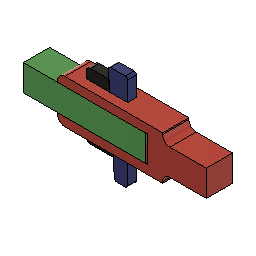
cotter and gip (Autodesk Fusion 360 design; units mm, degrees)
Autodesk Fusion 360 part; units mm, degrees
sketch "Sketch1" plane through (0, 0, 0) normal (0, 0, 1) x (1, 0, 0)
  line L0 (0, 0) -> (0, 20)
  line L1 (0, 20) -> (-170, 20)
  line L2 (-170, 20) -> (-170, -16)
  line L3 (-170, -16) -> (0, -16)
  line L4 (0, -16) -> (0, 0)
  line L5 (0, -16) -> (-39, -16)
  line L6 (83.0613, 20) -> (203.0613, 20)
  line L7 (203.0613, 20) -> (203.0613, -16)
  line L8 (203.0613, -16) -> (83.0613, -16)
  line L9 (83.0613, 20) -> (83.0613, 22)
  line L10 (83.0613, -16) -> (83.0613, -18)
  line L11 (83.0613, -28) -> (83.0613, -25)
  line L12 (93.0613, 32) -> (227.0613, 32)
  line L13 (227.0613, 32) -> (227.0613, 30)
  line L14 (227.0613, -28) -> (93.0613, -28)
  line L15 (237.0613, 20) -> (287.0613, 20)
  line L16 (237.0613, -16) -> (287.0613, -16)
  line L17 (287.0613, -16) -> (287.0613, 20)
  arc A0 (227.0613, 30) -> (237.0613, 20) centre (237.0613, 30) ccw
  line L18 (227.0613, -28) -> (227.0613, -26)
  arc A1 (237.0613, -16) -> (227.0613, -26) centre (237.0613, -26) ccw
  arc A2 (93.0613, 32) -> (83.0613, 22) centre (93.0613, 22) ccw
  arc A3 (83.0613, -18) -> (93.0613, -28) centre (93.0613, -18) ccw
  point P0 (83.0613, 32)
  point P1 (227.0613, 20)
  point P2 (227.0613, -16)
  dimension "d1" = 36
  dimension "d2" = 170
  dimension "d3" = 39
  dimension "d11" = 36
  dimension "d13" = 120
  dimension "d14" = 36
  dimension "d15" = 12
  dimension "d16" = 12
  dimension "d17" = 144
  dimension "d18" = 60
  dimension "d20" = 60
  dimension "d21" = 10
  dimension "d22" = 10
  dimension "d23" = 10
  dimension "d24" = 10
  constraint coincident L0.start L4.end
  constraint vertical L0
  constraint perpendicular L0 L1
  constraint perpendicular L1 L2
  constraint perpendicular L2 L3
  constraint perpendicular L3 L4
  constraint coincident L3 L5.end
  constraint perpendicular L6 L7
  constraint perpendicular L6 L9
  constraint perpendicular L8 L10
  constraint coincident L10 L11.end
  constraint perpendicular L9 L12
  constraint perpendicular L12 L13
  constraint perpendicular L10 L14
  constraint coincident L13 P1
  constraint perpendicular L13 L15
  constraint coincident L13 P2
  constraint perpendicular L13 L16
  constraint perpendicular L15 L17
  constraint coincident L14.start L13
  constraint coincident P1 L15
  constraint tangent L13 A0
  constraint tangent L15 A0
  constraint coincident P2 L18
  constraint coincident P2 L16
  constraint tangent L18 A1
  constraint tangent L16 A1
  constraint coincident P0 L9
  constraint coincident P0 L12
  constraint tangent L9 A2
  constraint tangent L12 A2
  constraint coincident L11.start L10
  constraint tangent L10 A3
  constraint tangent L14 A3
  measures "d1" distance of L1.end L2.end
  measures "d2" distance of L0.end L1.end
  measures "d3" distance of L3.end L5.end
  measures "d11" distance of L8.end L6.start
  measures "d13" distance of L6.start L6.end
  measures "d14" distance of L6.end L7.end
  measures "d15" distance of L6.start P0
  measures "d16" distance of L8.end L11.start
  measures "d17" distance of P0 L12.end
  measures "d18" distance of L12.end L14.start
  measures "d20" distance of P2 L16.end
  measures "d21" radius of A0
  measures "d22" radius of A1
  measures "d23" radius of A2
  measures "d24" radius of A3
extrude "Extrude1" add sketch "Sketch1" along normal mid plane 36 makes body 1 at (-113.3333, -16, 6) makes body 2 at (270.3947, -4, 18)
sketch "Sketch2" plane through (0, 20, 0) normal (0, 1, 0) x (-1, 0, 0)
  line L0 (170, -18) -> (170, 18)
  line L1 (170, 18) -> (0, 18)
  line L2 (0, 18) -> (0, -18)
  line L3 (0, -18) -> (170, -18)
  line L4 (0, 18) -> (170, 18)
  line L5 (170, -18) -> (170, 18)
  line L6 (170, -18) -> (0, -18)
  line L7 (0, -18) -> (0, 18)
  line L8 (-227.0613, 18) -> (-93.0613, 18)
  line L9 (-93.0613, -18) -> (-93.0613, 18)
  line L10 (-93.0613, -18) -> (-227.0613, -18)
  line L11 (-227.0613, -18) -> (-227.0613, 18)
  line L12 (39, -6) -> (39, 6)
  line L13 (39, 6) -> (84, 6)
  line L14 (84, 6) -> (84, -6)
  line L15 (84, -6) -> (39, -6)
  line L16 (-93.0613, -18) -> (-122.0613, -18)
  line L17 (-122.0613, -18) -> (-122.0613, -6)
  line L18 (-122.0613, -6) -> (-122.0613, 6)
  line L19 (-122.0613, 6) -> (-167.0613, 6)
  line L20 (-167.0613, 6) -> (-167.0613, -6)
  line L21 (-167.0613, -6) -> (-122.0613, -6)
  dimension "d29" = 12
  dimension "d30" = 45
  dimension "d31" = 12
  dimension "d32" = 29
  dimension "d33" = 12
  dimension "d34" = 12
  dimension "d35" = 45
  dimension "d36" = 12
  constraint perpendicular L13 L14
  constraint coincident L9.start L10.start
  constraint perpendicular L9 L16
  constraint perpendicular L10 L17
  constraint parallel L17 L18
  constraint perpendicular L17 L19
  constraint perpendicular L19 L20
  measures "d29" distance of L12.start L12.end
  measures "d30" distance of L12.end L13.end
  measures "d31" distance of L13.end L14.end
  measures "d32" distance of L9.start L16.end
  measures "d33" distance of L16.end L17.end
  measures "d34" distance of L17.end L18.end
  measures "d35" distance of L18.end L19.end
  measures "d36" distance of L19.end L20.end
extrude "Extrude2" cut sketch "Sketch2" along normal blind 50 and the other way blind 80 contours L12 L13 L14 L15 | L18 L19 L20 L21 bodies 1 2
sketch "Sketch3" plane through (0, 0, 0) normal (0, 0, 1) x (1, 0, 0)
  line L0 (-92.1013, 37.2076) -> (-92.1013, 46.2076)
  line L1 (-92.1013, -31.7924) -> (-92.1013, -22.7924)
  line L2 (-92.1013, -22.7924) -> (-80.1013, -22.7924)
  line L3 (-80.1013, -22.7924) -> (-80.1013, 37.2076)
  line L4 (-80.1013, 37.2076) -> (-92.1013, 37.2076)
  arc A0 (-86.1013, 52.2076) -> (-92.1013, 46.2076) centre (-86.1013, 46.2076) ccw
  arc A1 (-92.1013, -31.7924) -> (-86.1013, -37.7924) centre (-86.1013, -31.7924) ccw
  line L5 (-35.1013, 70.3547) -> (-35.1013, -55.6453)
  line L6 (-38.1013, -58.6453) -> (-50.2989, -58.6453)
  line L7 (-38.1013, 73.3547) -> (-58.8898, 73.3547)
  line L8 (-61.8829, 70.1507) -> (-53.2919, -55.8493)
  arc A2 (-58.8898, 73.3547) -> (-61.8829, 70.1507) centre (-58.8898, 70.3547) ccw
  arc A3 (-35.1013, 70.3547) -> (-38.1013, 73.3547) centre (-38.1013, 70.3547) ccw
  arc A4 (-38.1013, -58.6453) -> (-35.1013, -55.6453) centre (-38.1013, -55.6453) ccw
  arc A5 (-53.2919, -55.8493) -> (-50.2989, -58.6453) centre (-50.2989, -55.6453) ccw
  line L9 (62.437, 7.3547) -> (-190, 7.3547) construction
  line L10 (-86.1013, 52.2076) -> (-60.6595, 52.2076)
  line L11 (-35.1013, 52.2076) -> (-35, 52.2076)
  line L12 (-35, -37.7924) -> (-35.1013, -37.7924)
  line L13 (-54.5231, -37.7924) -> (-86.1013, -37.7924)
  line L14 (-54.5231, -37.7924) -> (-60.6595, 52.2076)
  point P0 (-92.1013, 52.2076)
  point P1 (-92.1013, -37.7924)
  point P2 (-35.1013, 73.3547)
  point P3 (-35.1013, -58.6453)
  point P4 (-53.1013, -58.6453)
  point P5 (-62.1013, 73.3547)
  dimension "d41" = 15
  dimension "d42" = 15
  dimension "d43" = 60
  dimension "d44" = 12
  dimension "d45" = 12
  dimension "d47" = 6
  dimension "d48" = 6
  dimension "d49" = 132
  dimension "d50" = 18
  dimension "d51" = 27
  dimension "d52" = 3
  dimension "d53" = 3
  dimension "d54" = 3
  dimension "d55" = 3
  dimension "d56" = 90
  dimension "d58" = 66
  dimension "d75" = 45
  constraint vertical L0
  constraint perpendicular L0 L10
  constraint perpendicular L1 L12
  constraint perpendicular L1 L2
  constraint perpendicular L0 L4
  constraint perpendicular L2 L3
  constraint coincident P0 L10
  constraint coincident P0 L0
  constraint tangent A0 L10
  constraint tangent L0 A0
  constraint coincident P1 L1
  constraint coincident P1 L12
  constraint tangent L1 A1
  constraint tangent A1 L12
  constraint perpendicular L5 L10
  constraint perpendicular L5 L6
  constraint perpendicular L5 L7
  constraint coincident P5 L8
  constraint coincident P5 L7
  constraint tangent L8 A2
  constraint tangent L7 A2
  constraint coincident P2 L7
  constraint coincident P2 L5
  constraint tangent L7 A3
  constraint tangent L5 A3
  constraint coincident P3 L5
  constraint coincident P3 L6
  constraint tangent L5 A4
  constraint tangent L6 A4
  constraint coincident P4 L6
  constraint coincident P4 L8
  constraint tangent L6 A5
  constraint tangent L8 A5
  constraint perpendicular L5 L9
  constraint coincident L8 L10.end
  constraint coincident L5 L11.start
  constraint collinear L10 L11
  constraint coincident L5 L12.end
  constraint coincident L8 L13.start
  constraint collinear L12 L13
  measures "d41" distance of P1 L1.end
  measures "d42" distance of L0.start P0
  measures "d43" distance of L2 L4
  measures "d44" distance of L0.start L3.end
  measures "d45" distance of L1.end L2.end
  measures "d47" radius of A0
  measures "d48" radius of A1
  measures "d49" distance of P2 P3
  measures "d50" distance of P3 P4
  measures "d51" distance of P2 P5
  measures "d52" radius of A2
  measures "d53" radius of A3
  measures "d54" radius of A4
  measures "d55" radius of A5
  measures "d56" distance of L11.end L12.start
  measures "d58" distance of L7 L9
  measures "d75" distance of L3 L5
extrude "Extrude3" add sketch "Sketch3" along normal mid plane 12 separate body contours L5 L6 L7 L8 A2 A3 A4 A5 L14 makes body 3
move_body "Move1" bodies 3 to x (1, 0, 0) y (0, 1, 0) z (0, 0, 1) at (60, 0, 0)
extrude "Extrude4" add sketch "Sketch3" along normal mid plane 12 separate body contours L0 L1 L2 L3 L4 A0 A1 L8 L10 L13 L14 makes body 4
copy_body "Body->Comp1" bodies 1 removing the originals makes body 5 in component "Component"
copy_body "Body->Comp2" bodies 2 removing the originals makes body 6 in component "Component'"
copy_body "Body->Comp3" bodies 3 removing the originals makes body 7 in component "gip"
copy_body "Body->Comp4" bodies 4 removing the originals makes body 8 in component "cotter"
component "Component" placed x (1, 0, 0) y (0, 1, 0) z (0, 0, 1) at (34.1863, 109.6996, -7.9078)
component "Component'" placed x (1, 0, 0) y (0, 1, 0) z (0, 0, 1) at (-171.875, 109.6996, -7.9078)
component "gip" placed x (1, 0, 0) y (0, 1, 0) z (0, 0, 1) at (-29.7124, 98.3449, -7.9078)
component "cotter" placed x (1, 0, 0) y (0, 1, 0) z (0, 0, 1) at (30.2876, 104.492, -7.9078)
named bodies: "gip", "cotter"
